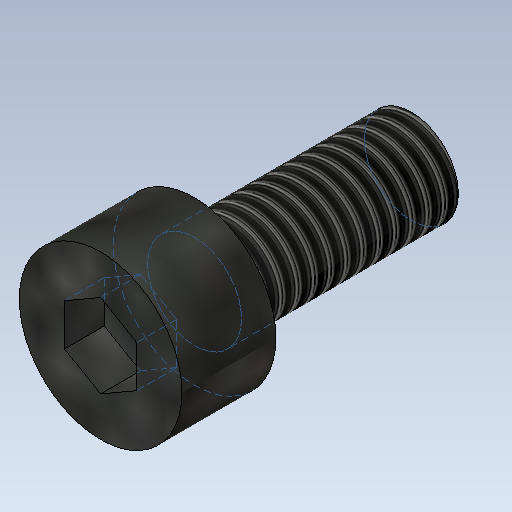
# Autodesk Inventor part: m2.6 6mm キャップボルト
Saved by Autodesk Inventor 2020 (Build 240168000, 168)
## iProperties
Part Number: m2.6 6mm キャップボルト
Material: 鋼
Document SubType Name: Modeling
Designer: 瑛飛
Density: 7.85 g/cm^3
Appearance: プレート
Mass: 0.544762 g
Surface Area: 1.25195 cm^2
Volume: 0.0693965 cm^3
Author: 瑛飛
Autodesk Inventor part; units mm, degrees
ref_plane "YZ Plane" through (0, 0, 0) normal (1, 0, 0) x (0, 1, 0)
ref_plane "XZ Plane" through (0, 0, 0) normal (0, 1, 0) x (-1, 0, 0)
ref_plane "XY Plane" through (0, 0, 0) normal (0, 0, 1) x (1, 0, 0)
sketch "スケッチ1" plane through (0, 0, 0) normal (0, 0, 1) x (1, 0, 0)
  circle A0 centre (0, 0) radius 1.3
  dimension "d0" = 2.6
  constraints: 1 centre point, 1 coincident
  measures "d0" diameter of A0
extrude "押し出し1" add sketch "スケッチ1" along normal blind 6
sketch "スケッチ2" plane through (0, 0, 6) normal (0, 0, 1) x (1, 0, 0)
  circle A0 centre (0, 0) radius 1.3 projected
  circle A1 centre (0, 0) radius 2.25
  dimension "d3" = 4.5
  constraints: 1 centre point, 1 coincident
  measures "d3" diameter of A1
extrude "押し出し2" add sketch "スケッチ2" along normal blind 2.6 contours A0 | A1
sketch "スケッチ3" plane through (0, 0, 8.6) normal (0, 0, 1) x (1, 0, 0)
  circle A0 centre (0, 0) radius 2.25 projected
  circle A1 centre (0, 0) radius 1.3 projected
  line L0 (0, 1.1547) -> (1, 0.5774)
  line L1 (1, 0.5774) -> (1, -0.5774)
  line L2 (1, -0.5774) -> (0, -1.1547)
  line L3 (0, -1.1547) -> (-1, -0.5774)
  line L4 (-1, -0.5774) -> (-1, 0.5774)
  line L5 (-1, 0.5774) -> (0, 1.1547)
  dimension "d6" = 2
  constraints: 12 end point, 1 coincident, 13 other
  measures "d6" distance between parallel lines of L3 L0
extrude "押し出し3" cut sketch "スケッチ3" against normal blind 1.1 contours L0 L1 L2 L3 L4 L5
thread "ねじ1" size "M2.6x0.45" class "6g" standard "ANSI Metric M Profile" full length
